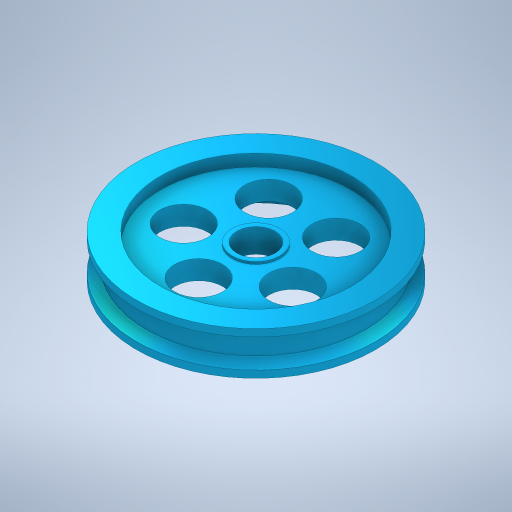
# Autodesk Inventor part: Pulley lớn
Saved by Autodesk Inventor 2023 (Build 270158000, 158)
## iProperties
Created: 2023-10-04
Part Number: Pulley lớn
Material: Iron, Cast
Document SubType Name: Modeling
Designer: huy20
Density: 7.15 g/cm^3
Appearance: Iron Gray
Author: huy20
Autodesk Inventor part; units mm, degrees
ref_plane "YZ Plane" through (0, 0, 0) normal (1, 0, 0) x (0, 1, 0)
ref_plane "XZ Plane" through (0, 0, 0) normal (0, 1, 0) x (-1, 0, 0)
ref_plane "XY Plane" through (0, 0, 0) normal (0, 0, 1) x (1, 0, 0)
sketch "Sketch1" plane through (0, 0, 0) normal (0, 0, 1) x (1, 0, 0)
  line L0 (-1.283, 24.9016) -> (-1.283, -22.4465)
  line L1 (23.717, 4.5) -> (23.717, -4.5)
  line L2 (23.717, -4.5) -> (18.717, -4.5)
  line L3 (18.717, -4.5) -> (18.717, -2)
  line L4 (18.717, -2) -> (2.717, -2)
  line L5 (23.717, 4.5) -> (18.717, 4.5)
  line L6 (18.717, 4.5) -> (18.717, 2)
  line L7 (18.717, 2) -> (2.717, 2)
  line L8 (2.717, 2) -> (2.717, -2)
  line L9 (23.717, 3) -> (21.717, 1.8453)
  line L10 (21.717, 1.8453) -> (21.717, -1.8453)
  line L11 (21.717, -1.8453) -> (23.717, -3)
  point P0 (0, 0)
  point P1 (18.717, 3.25)
  point P2 (18.717, -3.25)
  point P3 (2.717, 0)
  dimension "d0" = 50
  dimension "d1" = 8
  dimension "d2" = 5
  dimension "d3" = 9
  dimension "d4" = 1.5
  dimension "d5" = 1.5
  dimension "d6" = 60
  dimension "d7" = 2
  dimension "d20" = 4
  constraints: 24 end point, 6 perpendicular, 3 midpoint, 3 vertical, 2 equal length, 2 point on line, 1 horizontal, 1 horizontal alignment, 1 vertical alignment
  measures "d0" diameter of L1 L0
  measures "d1" diameter of L8 L0
  measures "d2" distance of L1.start L5.end
  measures "d3" distance between parallel lines of L2 L5
  measures "d4" distance of L1.start L9.start
  measures "d5" distance of L1.end L11.end
  measures "d6" angle of L1 L9
  measures "d7" distance between parallel lines of L1 L10
  measures "d20" distance between parallel lines of L4 L7
revolve "Revolution1" add sketch "Sketch1" angle 360 about axis through (-1.283, 24.9016, 0) along (0, -1, 0) contours L1 L9 L10 L11 L2 L3 L4 L8 L7 L6 L5
sketch "Sketch2" plane through (-1.283, 2, 0) normal (0, 1, 0) x (1, 0, 0)
  circle A0 centre (0, 0) radius 12 construction
  circle A1 centre (0, -12) radius 5
  circle A2 centre (11.4127, -3.7082) radius 5
  circle A3 centre (0, 0) radius 12 construction
  circle A4 centre (7.0534, 9.7082) radius 5
  circle A5 centre (0, 0) radius 12 construction
  circle A6 centre (-7.0534, 9.7082) radius 5
  circle A7 centre (0, 0) radius 12 construction
  circle A8 centre (-11.4127, -3.7082) radius 5
  circle A9 centre (0, 0) radius 12 construction
  point P0 (1.283, 0)
  dimension "d9" = 24
  dimension "d10" = 10
  dimension "d13" = 360
  constraints: 5 centre point, 2 coincident, 1 vertical alignment, 33 other
  measures "d10" diameter of A1
extrude "Extrusion1" cut sketch "Sketch2" against normal through all
sketch "Sketch3" plane through (-1.283, 2, 0) normal (0, 1, 0) x (1, 0, 0)
  circle A0 centre (0, 0) radius 5
  circle A1 centre (0, 0) radius 4
  point P0 (1.283, 0)
  dimension "d17" = 10
  constraints: 2 centre point, 1 coincident
  measures "d17" diameter of A0
extrude "Extrusion2" add sketch "Sketch3" along normal blind 0.5
mirror "Mirror1" about plane through (0, 0, 0) normal (0, 1, 0) of "Extrusion2"
body "Solid1"
